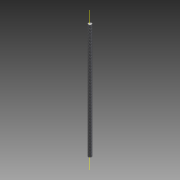
# Autodesk Inventor part: ASME Threaded Rod
Saved by Autodesk Inventor 2013 (Build 170138000, 138)
## iProperties
Created: 2013-01-17
Part Number: ASME Threaded Rod
Material: Steel
Document SubType Name: Modeling
Designer: actoennies
Density: 7.85 g/cm^3
Mass: 454.646 g
Surface Area: 184.948 cm^2
Volume: 57.9167 cm^3
Author: actoennies
Autodesk Inventor part; units mm, degrees
ref_plane "YZ Plane" through (0, 0, 0) normal (1, 0, 0) x (0, 1, 0)
ref_plane "XZ Plane" through (0, 0, 0) normal (0, 1, 0) x (-1, 0, 0)
ref_plane "XY Plane" through (0, 0, 0) normal (0, 0, 1) x (1, 0, 0)
sketch "Sketch1" plane through (0, 0, 0) normal (0, 1, 0) x (-1, 0, 0)
  circle A0 centre (0, 0) radius 6.35
  dimension "d0" = 12.7
  constraints: 1 centre point, 1 coincident
  measures "d0" diameter of A0
extrude "Extrusion1" add sketch "Sketch1" along normal blind 457.2
thread "Thread1" size "1-10 UNS" class "2A" standard "ANSI Unified Screw Threads" full length
body "Solid1"
